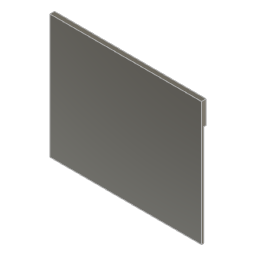
FLASHFORGECREATOR3 v3 (Autodesk Fusion 360 design; units mm, degrees)
Autodesk Fusion 360 part; units mm, degrees
sketch "Sketch1" plane through (0, 0, 0) normal (0, 0, 1) x (1, 0, 0)
  line L0 (0, 0) -> (330, 0)
  line L1 (330, 0) -> (330, 270)
  line L2 (330, 270) -> (0, 270)
  line L3 (0, 270) -> (0, 0)
  line L4 (0, 0) -> (330, 0)
  line L5 (330, 0) -> (330, 50)
  line L6 (330, 50) -> (0, 50)
  line L7 (0, 50) -> (0, 0)
  line L8 (0, 0) -> (330, 0) construction
  line L9 (330, 0) -> (330, 50) construction
  line L10 (330, 50) -> (0, 50) construction
  line L11 (0, 50) -> (0, 0) construction
  dimension "d1" = 330
  dimension "d2" = 270
  dimension "d3" = 50
  dimension "d8" = 20
  text T0 "TUTAJ NIE DRUKOWAĆ" font "Arial" height 20 bold align centre middle in box 330 x 50 at (0, 0) x (1, 0) y (0, 1) spacing 1 kerned
  constraint horizontal L0
  constraint vertical L1
  constraint horizontal L2
  constraint vertical L3
  constraint coincident L0.start L3.end
  constraint horizontal L4
  constraint vertical L5
  constraint horizontal L6
  constraint vertical L7
  constraint coincident L0.start
  constraint coincident L5.end
  measures "d1" distance of L0.start L0.end
  measures "d2" distance of L0.start L2.end
  measures "d3" distance of L0.start L6.end
extrude "Extrude1" add sketch "Sketch1" along normal blind 5 contours L1 L2 L3 L6
extrude "Extrude2" add sketch "Sketch1" along normal blind 10 contours L0 L1 L3 L4 L5 L6 L7
extrude "Extrude3" cut sketch "Sketch1" against normal blind 2 from surface at 10 text T0
move_body "Move1" bodies 1 to x (1, 0, 0) y (0, 0, -1) z (0, 1, 0) at (-165, 0, 0)
move_body "Move2" bodies 1 to x (1, 0, 0) y (0, 1, 0) z (0, 0, 1) at (0, 0, 135)
move_body "Move3" bodies 1 to x (1, 0, 0) y (0, 1, 0) z (0, 0, 1) at (0, -10, 0)
move_body "Move4" bodies 1 to x (1, 0, 0) y (0, 1, 0) z (0, 0, 1) at (0, -0.1, 0)
move_body "Move5" bodies 1 to x (1, 0, 0) y (0, 1, 0) z (0, 0, 1) at (0, 0.4, 0)
